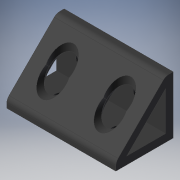
# Autodesk Inventor part: 30-4134 Aluminum
Saved by Autodesk Inventor 2019 (Build 230136000, 136)
## iProperties
Created: 2023-03-27
Part Number: 30-4134 Aluminum
Material: Generic
Catalog Web Link: www.cadenas.de
Description: 25-4134, 40-4334, 30-4134, 45-4334 25-4134-Black, 40-4334-Black, 30-4134-Black, 45-4334-Black-4 Hole Inside Gusset Corner Bracket
Vendor: 8020
Document SubType Name: Modeling
Designer: psAdmin
Manufacturer: 8020
Mass: 17.9479 g
Surface Area: 102.429 cm^2
Volume: 17.9479 cm^3
Density: 1 g/cm^3
Appearance: PSOLRGB-191-191-191
Category: PARTsolutions
Company: 8020
Title: 30-4134
Author: Cadenas PARTsolutions
Comments: 4 Hole Inside Gusset Corner Bracket
PSOL_IDENT_0: {$CADENAS_DATA/23d-libs/8020/metric/joining_plates/25_4134.prj},241 {VTYP=3D},{NB=30-4134},{LINA=30-
PSOL_IDENT_1: 4134},{NN=25-4134, 40-4334, 30-4134, 45-4334 25-4134-Black, 40-4334-Black, 30-4134-Black, 45-4334-Bl
PSOL_IDENT_2: ack},{DATE=31.07.2020 09:21:28},{GEOMDATE=15.01.2019 16:04:00},{VERSION=},{LINEID=30},{WBVAR=},{WBNU
PSOL_IDENT_3: MERIC=}  {NB=30-4134},{LINA=30-4134},{KT=DUMMY},{PN=30-4134},{SERIES=30},{MATERIAL=Aluminum},{GRADE=
PSOL_IDENT_4: 6105-T5},{FINISH=Clear Anodize},{A=57.00},{B=30.00},{C=30.00},{D=15.00},{E=12.70},{F=6.81},{G=30.00}
PSOL_IDENT_5: ,{H=13.50},{T=4.00},{W=.048},{A1=13.5000},{C2=15.000},{D1=4.000},{C3=12.700},{COLOR=.75,.75,.75}
NB: 30-4134
NN: 25-4134, 40-4334, 30-4134, 45-4334 25-4134-Black, 40-4334-Black, 30-4134-Black, 45-4334-Black
NT: 4 Hole Inside Gusset Corner Bracket
NBSYN: $PN.
LINA: 30-4134
CATALOG: 80/20
PN: 30-4134
SERIES: 30
MATERIAL: Aluminum
GRADE: 6105-T5
FINISH: Clear Anodize
A: 57
B: 30
C: 30
D: 15
E: 12.7
F: 6.81
G: 30
H: 13.5
T: 4
W: .048
SUPPLIER: 8020
ARTICLENO: 30-4134
BOMINFO: 30-4134
CREATOR: CADENAS GmbH
Autodesk Inventor part; units mm, degrees
ref_plane "YZ Plane" through (0, 0, 0) normal (1, 0, 0) x (0, 1, 0)
ref_plane "XZ Plane" through (0, 0, 0) normal (0, 1, 0) x (-1, 0, 0)
ref_plane "XY Plane" through (0, 0, 0) normal (0, 0, 1) x (1, 0, 0)
sketch "Sketch_1" plane through (0, 0, 0) normal (1, 0, 0) x (0, 1, 0)
  line L0 (2.3431, 30) -> (0, 30)
  line L1 (0, 30) -> (0, 0)
  line L2 (0, 0) -> (30, 0)
  line L3 (30, 0) -> (30, 2.3431)
  arc A0 (30, 2.3431) -> (28.8284, 5.1716) centre (26, 2.3431) ccw
  line L4 (28.8284, 5.1716) -> (5.1716, 28.8284)
  arc A1 (5.1716, 28.8284) -> (2.3431, 30) centre (2.3431, 26) ccw
  line L5 (4, 24.3431) -> (4, 4)
  line L6 (4, 4) -> (24.3431, 4)
  line L7 (24.3431, 4) -> (4, 24.3431)
  constraints: 16 end point, 4 point on circle, 2 centre point
extrude "Extrusion1" add sketch "Sketch_1" along normal mid plane 57
sketch "Sketch2" plane through (-28.5, 0, 0) normal (0, -1, 0) x (1, 0, 0)
  point P0 (43.5, 15)
hole "Hole1" at (15, 0, 15) direction (0, 1, 0) diameter 6.81 depth 4
sketch "Sketch3" plane through (28.5, 30, 0) normal (0, 0, -1) x (-1, 0, 0)
  point P0 (13.5, -15)
hole "Hole2" at (15, 15, 0) direction (0, 0, 1) diameter 6.81 depth 4
sketch "Sketch_4" plane through (0, 0, 30) normal (0, 0, 1) x (1, 0, 0)
  circle A0 centre (15, 15) radius 6.35
  constraints: 1 centre point
extrude "Extrusion2" cut sketch "Sketch_4" against normal blind 26
sketch "Sketch_5" plane through (0, 30, 0) normal (0, 1, 0) x (1, 0, 0)
  circle A0 centre (15, -15) radius 6.35
  constraints: 1 centre point
extrude "Extrusion3" cut sketch "Sketch_5" against normal blind 26
sketch "Sketch6" plane through (28.5, 30, 0) normal (0, 0, -1) x (-1, 0, 0)
  point P0 (43.5, -15)
hole "Hole3" at (-15, 15, 0) direction (0, 0, 1) diameter 6.81 depth 4
sketch "Sketch7" plane through (-28.5, 0, 0) normal (0, -1, 0) x (1, 0, 0)
  point P0 (13.5, 15)
hole "Hole4" at (-15, 0, 15) direction (0, 1, 0) diameter 6.81 depth 4
sketch "Sketch_8" plane through (0, 30, 0) normal (0, 1, 0) x (1, 0, 0)
  circle A0 centre (-15, -15) radius 6.35
  constraints: 1 centre point
extrude "Extrusion4" cut sketch "Sketch_8" against normal blind 26
sketch "Sketch_9" plane through (0, 0, 30) normal (0, 0, 1) x (1, 0, 0)
  circle A0 centre (-15, 15) radius 6.35
  constraints: 1 centre point
extrude "Extrusion5" cut sketch "Sketch_9" against normal blind 26
body "Solid1"
